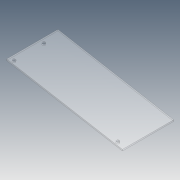
# Autodesk Inventor part: GE-12086-03
Saved by Autodesk Inventor 2012 (Build 160160000, 160)
## iProperties
Created: 2011-10-10
Part Number: GE-12086-03
Document SubType Name: Modeling
Designer: dfoster
Density: 1 g/cm^3
Description: Top
Material: Default
Title: Top
Author: dfoster
Autodesk Inventor part; units mm, degrees
ref_plane "YZ Plane" through (0, 0, 0) normal (1, 0, 0) x (0, 1, 0)
ref_plane "XZ Plane" through (0, 0, 0) normal (0, 1, 0) x (-1, 0, 0)
ref_plane "XY Plane" through (0, 0, 0) normal (0, 0, 1) x (1, 0, 0)
sketch "Sketch1" plane through (0, 0, 0) normal (0, 0, 1) x (1, 0, 0)
  line L0 (-136.525, 26.9398) -> (153.9875, -24.2854) projected
  line L1 (153.9875, -21.0615) -> (153.9875, -24.2854) projected
  line L2 (153.9875, -21.0615) -> (-136.525, 30.1637) projected
  line L3 (-136.525, 26.9398) -> (-136.525, 30.1637) projected
  point P0 (0, 0)
extrude "Extrusion1" add sketch "Sketch1" along normal blind 117.475
hole "Hole1" at (-127.1447, 28.5097, 109.5375) direction (-0.1736, -0.9848, 0) diameter 6.731 depth 25.4 tip angle 118
pattern_linear "Rectangular Pattern1" count 2 spacing 68.2625 along (0, 0, -1) of "Hole1"
pattern_linear "Rectangular Pattern2" count 2 spacing 241.3 along (0.9848, -0.1736, 0) of "Hole1"
body "Solid1"
